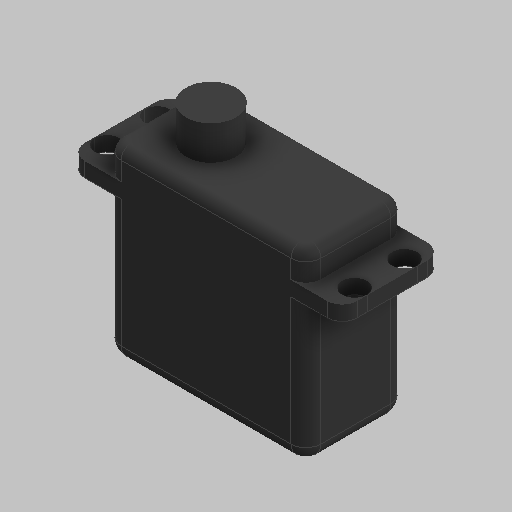
# Autodesk Inventor part: Feedback 360
Saved by Autodesk Inventor 2025 (Build 290162010, 162A)
## iProperties
Created: 2024-06-08
Part Number: Feedback 360
Material: Genérico
Document SubType Name: Sheet Metal
Designer: juesr
Density: 1 g/cm^3
Sheet Metal Rule: Por defecto_mm
Appearance: Valor por defecto
Author: juesr
Autodesk Inventor part; units mm, degrees
ref_plane "YZ Plane" through (0, 0, 0) normal (1, 0, 0) x (0, 1, 0)
ref_plane "XZ Plane" through (0, 0, 0) normal (0, 1, 0) x (-1, 0, 0)
ref_plane "XY Plane" through (0, 0, 0) normal (0, 0, 1) x (1, 0, 0)
sketch "Boceto1" plane through (0, 0, 0) normal (0, 1, 0) x (-1, 0, 0)
  line L0 (20, 10) -> (-20, 10)
  line L1 (-20, 10) -> (-20, -10)
  line L2 (-20, -10) -> (20, -10)
  line L3 (20, -10) -> (20, 10)
  point P0 (0, 0)
  point P1 (-20, 0)
  dimension "d0" = 20
  dimension "d1" = 40
  dimension "d2" = 10
  dimension "d3" = 20
  constraints: 8 end point, 2 parallel, 1 horizontal, 1 midpoint, 1 perpendicular
  measures "d0" distance between parallel lines of L2 L0
  measures "d1" distance from line of point (-20, 0) L3
  measures "d2" distance from line of L2 point (0, 0)
  measures "d3" distance from line of L1 point (0, 0)
extrude "Extrusión1" add sketch "Boceto1" along normal blind 28.5
fillet "Empalme1" radius 3 4 edges at (0, 0, 10) (20, 0, 0) (0, 0, -10) (-20, 0, 0)
fillet "Empalme2" radius 3 6 edges at (-20, 15.75, -10) (-19.1213, 0.8787, -9.1213) (-20, 15.75, 10) (-19.1213, 0.8787, 9.1213) (20, 15.75, 10) (19.1213, 0.8787, 9.1213)
fillet "Empalme3" radius 3 2 edges at (20, 15.75, -10) (19.1213, 0.8787, -9.1213)
sketch "Boceto2" plane through (0, 28.5, 0) normal (0, 1, 0) x (1, 0, 0)
  line L0 (-27.25, 10) -> (27.25, 10)
  line L1 (27.25, 10) -> (27.25, -10)
  line L2 (27.25, -10) -> (-27.25, -10)
  line L3 (-27.25, -10) -> (-27.25, 10)
  line L4 (17, 10) -> (-17, 10) projected
  line L5 (-17, -10) -> (17, -10) projected
  point P0 (0, 0)
  dimension "d9" = 0
  dimension "d10" = 0
  dimension "d11" = 54.5
  dimension "d12" = 27.25
  constraints: 8 end point, 2 parallel, 1 horizontal, 1 perpendicular
  measures "d9" distance between parallel lines of L4 L0
  measures "d10" distance between parallel lines of L5 L2
  measures "d11" distance between parallel lines of L1 L3
  measures "d12" distance from line of L1 point (0, 0)
extrude "Extrusión2" add sketch "Boceto2" along normal blind 3
fillet "Empalme4" radius 3 3 edges at (-27.25, 30, 10) (-27.25, 30, -10) (27.25, 30, 10)
fillet "Empalme5" radius 3 1 edges at (27.25, 30, -10)
sketch "Boceto3" plane through (0, 31.5, 0) normal (0, 1, 0) x (1, 0, 0)
  line L0 (-17, 10) -> (17, 10) projected
  line L1 (-24.25, -10) -> (24.25, -10) projected
  line L2 (-20, 10) -> (20, 10)
  line L3 (20, 10) -> (20, -10)
  line L4 (20, -10) -> (-20, -10)
  line L5 (-20, -10) -> (-20, 10)
  point P0 (0, 0)
  dimension "d17" = 20
  dimension "d18" = 20
  constraints: 8 end point, 2 parallel, 2 point on line, 1 horizontal, 1 perpendicular
  measures "d17" distance from line of point (0, 0) L3
  measures "d18" distance from line of point (0, 0) L5
extrude "Extrusión3" add sketch "Boceto3" along normal blind 5.7
fillet "Empalme6" radius 3 3 edges at (20, 34.35, -10) (20, 34.35, 10) (-20, 34.35, -10)
fillet "Empalme7" radius 2 7 edges at (-20, 37.2, 1.5) (-19.1213, 37.2, -9.1213) (0, 37.2, -10) (19.1213, 37.2, -9.1213) (20, 37.2, 0) (19.1213, 37.2, 9.1213) (-1.5, 37.2, 10)
fillet "Empalme8" radius 3 2 edges at (-20, 33.35, 10) (-19.4142, 36.6142, 9.4142)
sketch "Boceto4" plane through (0, 31.5, 0) normal (0, 1, 0) x (1, 0, 0)
  circle A0 centre (-24.75, 5) radius 2.5
  line L0 (-38.2556, 0) -> (37.7734, 0)
  line L1 (0, 20.4997) -> (0, -23.7455)
  circle A1 centre (-24.75, -5) radius 2.5
  circle A2 centre (24.75, 5) radius 2.5
  circle A3 centre (24.75, -5) radius 2.5
  point P0 (0, 0)
  dimension "d24" = 24.75
  dimension "d25" = 5
  dimension "d26" = 5
  dimension "d27" = 24.75
  constraints: 4 centre point, 4 end point, 3 symmetric about line, 1 horizontal, 1 vertical, 3 other
  measures "d24" horizontal distance of point (0, 0) A0.centre
  measures "d25" vertical distance of point (0, 0) A0.centre
  measures "d26" diameter of A0
  measures "d27" distance from line of L1 A2.centre
extrude "Extrusión4" cut sketch "Boceto4" against normal blind 5
sketch "Boceto5" plane through (0, 37.2, 0) normal (0, 1, 0) x (1, 0, 0)
  circle A0 centre (-9, 0) radius 5
  point P0 (0, 0)
  dimension "d30" = 10
  dimension "d31" = 9
  constraints: 1 centre point
  measures "d30" diameter of A0
  measures "d31" distance of point (0, 0) A0.centre
extrude "Extrusión5" add sketch "Boceto5" along normal blind 7
equation "\"Radio_pliegue\" = Grosor"
equation "\"Anchura_desahogo_plegado\" = Grosor"
equation "\"Profundidad_desahogo_plegado\" = 0.5 * Grosor"
equation "\"Tamaño_destalonado\" = 4 * Grosor"
equation "\"Remanente_mínimo\" = 2 * Grosor"
equation "\"Radiodetransición\" = Radio_pliegue"
equation "\"Tamaño_de_radio_de_Jacobi\" = Radio_pliegue"
equation "\"TamañoSeparación\" = Grosor"
equation "\"Grosor\" = 0.5"
